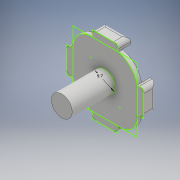
# Autodesk Inventor part: spider_support
Saved by Autodesk Inventor 2018 (Build 220112000, 112)
## iProperties
Created: 2018-09-20
Part Number: spider_support
Material: Generic
Document SubType Name: Modeling
Designer: ryanc
Density: 1 g/cm^3
Appearance: Default
Author: ryanc
Autodesk Inventor part; units mm, degrees
ref_plane "YZ Plane" through (0, 0, 0) normal (1, 0, 0) x (0, 1, 0)
ref_plane "XZ Plane" through (0, 0, 0) normal (0, 1, 0) x (-1, 0, 0)
ref_plane "XY Plane" through (0, 0, 0) normal (0, 0, 1) x (1, 0, 0)
sketch "Sketch1" plane through (0, 0, 0) normal (0, 1, 0) x (-1, 0, 0)
  circle A0 centre (0.1717, 0) radius 4.85
  line L0 (15, 15) -> (-15, 15)
  line L1 (-15, 15) -> (-15, -15)
  line L2 (-15, -15) -> (15, -15)
  line L3 (15, -15) -> (15, 15)
  line L4 (0, 15) -> (6, 15)
  line L5 (6, 15) -> (6, 18)
  line L6 (6, 18) -> (0, 18)
  line L7 (0, 18) -> (-6, 18)
  line L8 (-6, 18) -> (-6, 15)
  line L9 (-6, 15) -> (0, 15)
  line L10 (6, -15) -> (-6, -15)
  line L11 (-6, -15) -> (-6, -18)
  line L12 (-6, -18) -> (6, -18)
  line L13 (6, -18) -> (6, -15)
  line L14 (15, 6) -> (18, 6)
  line L15 (18, 6) -> (18, -6)
  line L16 (18, -6) -> (15, -6)
  line L17 (15, -6) -> (15, 6)
  line L18 (-15, -6) -> (-18, -6)
  line L19 (-18, -6) -> (-18, 6)
  line L20 (-18, 6) -> (-15, 6)
  line L21 (-15, 6) -> (-15, -6)
  arc A1 (15, 6) -> (6, 15) centre (6.5, 6.5) ccw
  arc A2 (6, -15) -> (15, -6) centre (4, -4) ccw
  arc A3 (-15, -6) -> (-6, -15) centre (-7, -7) ccw
  arc A4 (-6.3124, 15) -> (-15, 6) centre (-3.6523, 3.7392) ccw
  point P0 (0, 0)
  dimension "d0" = 9.7
  constraints: 44 end point, 10 parallel, 8 point on circle, 7 point on line, 6 horizontal, 6 perpendicular, 5 centre point, 1 midpoint
  measures "d0" diameter of A0
extrude "Extrusion1" add sketch "Sketch1" along normal blind 6 contours L0 L8 L7 L6 L5 | L14 L15 L16 L3 | L1 L18 L19 L20 | L13 L12 L11 L2
extrude "Extrusion2" cut sketch "Sketch1" along normal blind 3 contours L0 A1 L3 A2 L2 A3 L1 A4 | A1 L0 | A1 L3 | L1 A3 | A3 L2
extrude "Extrusion3" add sketch "Sketch1" along normal blind 2 contours A0 | L0 A1 L3 A2 L2 A3 L1 A4 | A1 L0 | A1 L3 | L1 A3 | A3 L2
fillet "Fillet1" radius 2 12 edges at (18, 3, -6) (6, 3, -18) (-6, 3, -18) (-18, 3, -6) (-18, 3, 6) (-6, 3, 18) (6, 3, 18) (18, 3, 6) (0, 6, 18) (-18, 6, 0) (0, 6, -18) (18, 6, 0)
extrude "Extrusion4" add sketch "Sketch1" against normal blind 20 contours A0
body "Solid1"
